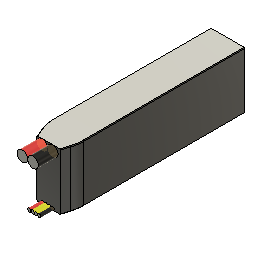
2024-11-05_development-hexapod-mounts (Autodesk Fusion 360 archive; units mm, degrees)
design "battery"
Autodesk Fusion 360 part; units mm, degrees
(part 1 of 2)
sketch "Sketch1" plane through (0, 0, 0) normal (0, 0, 1) x (1, 0, 0)
  line L0 (0, 0) -> (26, 0)
  line L1 (26, 0) -> (26, 137)
  line L2 (26, 137) -> (0, 137)
  line L3 (0, 137) -> (0, 0)
  dimension "d1" = 26
  dimension "d2" = 137
  constraint horizontal L0
  constraint vertical L1
  constraint horizontal L2
  constraint vertical L3
  constraint coincident L0.start L3.end
  measures "d1" distance of L0.start L0.end
  measures "d2" distance of L0.start L2.end
extrude "Extrude1" add sketch "Sketch1" along normal blind 43 makes body 1
sketch "Sketch2" plane through (0, 0, 0) normal (0, -1, 0) x (1, 0, 0)
  line L0 (0, 0) -> (26, 0)
  line L1 (26, 0) -> (26, 43)
  line L2 (26, 43) -> (0, 43)
  line L3 (0, 43) -> (0, 0)
  line L4 (21, 35) -> (5, 35) construction
  line L5 (5, 35) -> (5, 51) construction
  line L6 (5, 51) -> (21, 51) construction
  line L7 (21, 51) -> (21, 35) construction
  line L8 (21, 35) -> (5, 51) construction
  line L9 (5, 35) -> (21, 51) construction
  line L10 (13, 43) -> (5, 35) construction
  line L11 (13, 43) -> (21, 35) construction
  circle A0 centre (9, 39) radius 4
  circle A1 centre (17, 39) radius 4
  point P0 (13, 43)
  dimension "d5" = 16
  dimension "d6" = 16
  constraint horizontal L4
  constraint perpendicular L4 L5
  constraint parallel L4 L6
  constraint parallel L5 L7
  constraint coincident L8 P0
  constraint coincident L9 P0
  constraint midpoint L2 P0
  constraint coincident P0 L10.start
  constraint midpoint L10 A0.centre
  constraint tangent L2 A0
  constraint midpoint L11 A1.centre
  constraint tangent L2 A1
  measures "d5" distance of L5.end L6.end
  measures "d6" distance of L4.end L5.end
extrude "Extrude2" add sketch "Sketch2" along normal blind 15 separate body contours A0 | A1 makes body 2
sketch "Sketch3" plane through (0, 0, 0) normal (0, -1, 0) x (1, 0, 0)
  line L0 (0, 0) -> (26, 0)
  line L1 (26, 0) -> (26, 43)
  line L2 (26, 43) -> (0, 43)
  line L3 (0, 43) -> (0, 0)
  line L4 (18, 2.5) -> (8, 2.5) construction
  line L5 (8, 2.5) -> (8, -2.5) construction
  line L6 (8, -2.5) -> (18, -2.5) construction
  line L7 (18, -2.5) -> (18, 2.5) construction
  line L8 (18, 2.5) -> (8, -2.5) construction
  line L9 (8, 2.5) -> (18, -2.5) construction
  line L10 (8, 2.5) -> (8, 0)
  line L11 (8, 1.25) -> (9.25, 1.25) construction
  circle A0 centre (9.25, 1.25) radius 1.25
  circle A1 centre (11.75, 1.25) radius 1.25
  circle A2 centre (14.25, 1.25) radius 1.25
  circle A3 centre (16.75, 1.25) radius 1.25
  point P0 (13, 0)
  dimension "d9" = 10
  dimension "d10" = 5
  dimension "d11" = 1.25
  constraint horizontal L4
  constraint perpendicular L4 L5
  constraint parallel L4 L6
  constraint parallel L5 L7
  constraint coincident L8 P0
  constraint coincident L9 P0
  constraint midpoint L0 P0
  constraint midpoint L5 L10.end
  constraint midpoint L10 L11.start
  constraint perpendicular L5 L11
  constraint coincident L11.end A0.centre
  constraint tangent L4 A0
  measures "d9" distance of L5.end L6.end
  measures "d10" distance of L4.end L5.end
  measures "d11" distance of L11.start L11.end
extrude "Extrude3" add sketch "Sketch3" along normal blind 10 separate body contours A0 | A1 | A2 | A3 makes body 3
chamfer "Chamfer1" distance 3 distance2 10 1 edges at (26, 0, 21.5) measured on face at (8.6667, 0, 14.3333) on bodies 1
chamfer "Chamfer2" distance 12 distance2 5 1 edges at (0, 0, 21.5) measured on face at (0, 91.3333, 14.3333) on bodies 1
fillet "Fillet1" radius 30 2 edges at (0, 12, 21.5) (26, 10, 21.5) on bodies 1
chamfer "Chamfer3" distance 0.5 distance2 0.5 12 edges at (25.682, 10.0467, 0) (26, 75.7015, 0) (23.8674, 2.8913, 0) (0, 77.5, 0) (0.5826, 12.1165, 0) (3.6538, 3.2308, 0) (0.5826, 12.1165, 43) (0, 77.5, 43) (3.6538, 3.2308, 43) (26, 75.7015, 43) (23.8674, 2.8913, 43) (25.682, 10.0467, 43) 1 faces at (17.3333, 137, 14.3333) measured on face at (25.9843, 13.4317, 14.3333) measured on face at (26, 55.2687, 14.3333) measured on face at (23.5783, 1.9275, 14.3333) measured on face at (0, 97.3333, 14.3333) measured on face at (1.8284, 7.687, 28.6667) measured on face at (3.2051, 4.3077, 28.6667) measured on face at (1.8284, 7.687, 28.6667) measured on face at (17.3333, 56.4677, 43) measured on face at (3.2051, 4.3077, 28.6667) measured on face at (17.3333, 56.4677, 43) measured on face at (23.5783, 1.9275, 14.3333) measured on face at (25.9843, 13.4317, 14.3333) on bodies 1

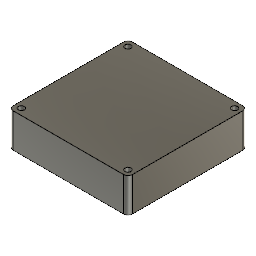
design "noctua_fan_80mm"
Autodesk Fusion 360 part; units mm, degrees
box "BoxPrimitive1" add length 80 width 80 height 23 placed x (0, -1, 0) y (1, 0, 0) z (0, 0, 1) at (0, 0, 0)
fillet "Fillet1" radius 3 4 edges at (0, -80, 11.5) (80, -80, 11.5) (80, 0, 11.5) (0, 0, 11.5)
sketch "Sketch2" plane through (0, 0, 23) normal (0, 0, 1) x (-1, 0, 0)
  arc A0 (-3, 0) -> (0, 3) centre (-3, 3) ccw
  line L0 (0, 3) -> (0, 77)
  arc A1 (0, 77) -> (-3, 80) centre (-3, 77) ccw
  line L1 (-3, 80) -> (-77, 80)
  arc A2 (-77, 80) -> (-80, 77) centre (-77, 77) ccw
  line L2 (-80, 77) -> (-80, 3)
  arc A3 (-80, 3) -> (-77, 0) centre (-77, 3) ccw
  line L3 (-77, 0) -> (-3, 0)
  circle A4 centre (-75.75, 75.75) radius 2
  circle A5 centre (-75.75, 4.25) radius 2
  circle A6 centre (-4.25, 75.75) radius 2
  circle A7 centre (-4.25, 4.25) radius 2
  dimension "d8" = 4
  dimension "d9" = 4
  dimension "d10" = 4
  dimension "d11" = 4
  dimension "d12" = 4.25
  dimension "d13" = 4.25
  dimension "d14" = 4.25
  dimension "d15" = 4.25
  dimension "d16" = 4.25
  dimension "d17" = 4.25
  dimension "d18" = 4.25
  dimension "d19" = 4.25
  measures "d8" diameter of A4
  measures "d9" diameter of A5
  measures "d10" diameter of A6
  measures "d11" diameter of A7
  measures "d12" distance of L1 A4.centre
  measures "d13" distance of L2 A4.centre
  measures "d14" distance of L3 A5.centre
  measures "d15" distance of L2 A5.centre
  measures "d16" distance of L3 A7.centre
  measures "d17" distance of L0 A7.centre
  measures "d18" distance of L1 A6.centre
  measures "d19" distance of L0 A6.centre
extrude "Extrude1" cut sketch "Sketch2" against normal blind 35 contours A4 | A5 | A6 | A7

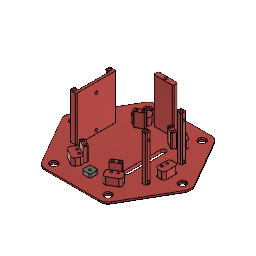
design "base"
Autodesk Fusion 360 part; units mm, degrees
sketch "Sketch1" plane through (0, 0, 0) normal (0, 0, 1) x (1, 0, 0)
  line L0 (130, 0) -> (65, 112.5833)
  line L1 (65, 112.5833) -> (-65, 112.5833)
  line L2 (-65, 112.5833) -> (-130, 0)
  line L3 (-130, 0) -> (-65, -112.5833)
  line L4 (-65, -112.5833) -> (65, -112.5833)
  line L5 (65, -112.5833) -> (130, 0)
  dimension "d1" = 130
  measures "d1" distance of L0.start origin
extrude "Extrude1" add sketch "Sketch1" along normal blind 6.5 makes body 1
fillet "Fillet1" radius 18 6 edges at (-130, 0, 3.25) (-65, -112.5833, 3.25) (65, -112.5833, 3.25) (130, 0, 3.25) (65, 112.5833, 3.25) (-65, 112.5833, 3.25) on bodies 1
chamfer "Chamfer2" distance 3.25 angle 45 12 edges at (0, -112.5833, 0) (63.6077, -110.1718, 0) (97.5, -56.2917, 0) (127.2154, 0, 0) (97.5, 56.2917, 0) (63.6077, 110.1718, 0) (0, 112.5833, 0) (-63.6077, 110.1718, 0) (-97.5, 56.2917, 0) (-127.2154, 0, 0) (-97.5, -56.2917, 0) (-63.6077, -110.1718, 0) on bodies 1
sketch "Sketch2" plane through (0, 0, 6.5) normal (0, 0, 1) x (-1, 0, 0)
  arc A0 (54.6077, -112.5833) -> (70.1962, -103.5833) centre (54.6077, -94.5833) ccw
  line L0 (70.1962, -103.5833) -> (124.8038, -9)
  arc A1 (124.8038, -9) -> (124.8038, 9) centre (109.2154, 0) ccw
  line L1 (124.8038, 9) -> (70.1962, 103.5833)
  line L2 (54.6077, 112.5833) -> (-54.6077, 112.5833)
  line L3 (-70.1962, 103.5833) -> (-124.8038, 9)
  arc A2 (-124.8038, 9) -> (-124.8038, -9) centre (-109.2154, 0) ccw
  line L4 (-124.8038, -9) -> (-70.1962, -103.5833)
  arc A3 (-70.1962, -103.5833) -> (-54.6077, -112.5833) centre (-54.6077, -94.5833) ccw
  line L5 (-54.6077, -112.5833) -> (54.6077, -112.5833)
  circle A4 centre (109.2154, 0) radius 7
  circle A5 centre (109.2154, 0) radius 6
  circle A6 centre (73.4654, -5) radius 2.25
  arc A7 (73.7154, 14.55) -> (68.7154, 9.55) centre (73.7154, 9.55) ccw
  line L6 (68.7154, 9.55) -> (68.7154, -9.55)
  circle A8 centre (73.4654, 5) radius 2.25
  line L7 (86.7154, 9.55) -> (86.7154, -9.55)
  line L8 (68.7154, 0) -> (86.7154, 0) construction
  arc A9 (68.7154, -9.55) -> (73.7154, -14.55) centre (73.7154, -9.55) ccw
  arc A10 (73.7154, 14.55) -> (68.7154, 9.55) centre (73.7154, 9.55) ccw
  line L9 (81.7154, 14.55) -> (73.7154, 14.55)
  line L10 (68.7154, 30.5204) -> (68.7154, -30.5204)
  line L11 (73.7154, -14.55) -> (81.7154, -14.55)
  line L12 (73.4654, 5) -> (68.7154, 5) construction
  line L13 (73.4654, -5) -> (68.7154, -5) construction
  line L14 (127.2154, 0) -> (-127.2154, 0) construction
  line L15 (0, -112.5833) -> (0, 112.5833) construction
  arc A11 (-124.8038, 9) -> (-124.8038, -9) centre (-109.2154, 0) ccw
  arc A12 (-70.1962, -103.5833) -> (-54.6077, -112.5833) centre (-54.6077, -94.5833) ccw
  arc A13 (54.6077, -112.5833) -> (70.1962, -103.5833) centre (54.6077, -94.5833) ccw
  arc A14 (81.7154, -14.55) -> (86.7154, -9.55) centre (81.7154, -9.55) ccw
  arc A15 (86.7154, 9.55) -> (81.7154, 14.55) centre (81.7154, 9.55) ccw
  circle A16 centre (32.4026, 66.1229) radius 2.25
  line L16 (26.0872, 64.2843) -> (42.6282, 54.7343)
  line L17 (34.3577, 59.5093) -> (43.3577, 75.0977) construction
  arc A17 (70.1962, 103.5833) -> (54.6077, 112.5833) centre (54.6077, 94.5833) ccw
  arc A18 (42.6282, 54.7343) -> (49.4584, 56.5644) centre (45.1282, 59.0644) ccw
  line L18 (41.0628, 61.1229) -> (38.6878, 57.0093) construction
  arc A19 (24.257, 71.1144) -> (26.0872, 64.2843) centre (28.5872, 68.6144) ccw
  line L19 (28.257, 78.0426) -> (24.257, 71.1144)
  circle A20 centre (41.0628, 61.1229) radius 2.25
  arc A21 (53.4584, 63.4926) -> (51.6282, 70.3227) centre (49.1282, 65.9926) ccw
  circle A22 centre (54.6077, 94.5833) radius 6
  circle A23 centre (54.6077, 94.5833) radius 7
  line L20 (32.4026, 66.1229) -> (30.0276, 62.0093) construction
  arc A24 (24.257, 71.1144) -> (26.0872, 64.2843) centre (28.5872, 68.6144) ccw
  line L21 (26.0872, 64.2843) -> (42.6282, 54.7343)
  line L22 (49.4584, 56.5644) -> (53.4584, 63.4926)
  line L23 (35.0872, 79.8727) -> (51.6282, 70.3227)
  arc A25 (35.0872, 79.8727) -> (28.257, 78.0426) centre (32.5872, 75.5426) ccw
  circle A26 centre (-41.0628, 61.1229) radius 2.25
  line L24 (-42.6282, 54.7343) -> (-26.0872, 64.2843)
  line L25 (-34.3577, 59.5093) -> (-43.3577, 75.0977) construction
  arc A27 (-54.6077, 112.5833) -> (-70.1962, 103.5833) centre (-54.6077, 94.5833) ccw
  arc A28 (-26.0872, 64.2843) -> (-24.257, 71.1144) centre (-28.5872, 68.6144) ccw
  line L26 (-32.4026, 66.1229) -> (-30.0276, 62.0093) construction
  arc A29 (-49.4584, 56.5644) -> (-42.6282, 54.7343) centre (-45.1282, 59.0644) ccw
  line L27 (-53.4584, 63.4926) -> (-49.4584, 56.5644)
  circle A30 centre (-32.4026, 66.1229) radius 2.25
  arc A31 (-28.257, 78.0426) -> (-35.0872, 79.8727) centre (-32.5872, 75.5426) ccw
  circle A32 centre (-54.6077, 94.5833) radius 6
  circle A33 centre (-54.6077, 94.5833) radius 7
  line L28 (-41.0628, 61.1229) -> (-38.6878, 57.0093) construction
  arc A34 (-49.4584, 56.5644) -> (-42.6282, 54.7343) centre (-45.1282, 59.0644) ccw
  line L29 (-42.6282, 54.7343) -> (-26.0872, 64.2843)
  line L30 (-24.257, 71.1144) -> (-28.257, 78.0426)
  line L31 (-51.6282, 70.3227) -> (-35.0872, 79.8727)
  arc A35 (-51.6282, 70.3227) -> (-53.4584, 63.4926) centre (-49.1282, 65.9926) ccw
  circle A36 centre (-73.4654, -5) radius 2.25
  line L32 (-68.7154, -9.55) -> (-68.7154, 9.55)
  line L33 (-68.7154, 0) -> (-86.7154, 0) construction
  arc A37 (-124.8038, 9) -> (-124.8038, -9) centre (-109.2154, 0) ccw
  arc A38 (-68.7154, 9.55) -> (-73.7154, 14.55) centre (-73.7154, 9.55) ccw
  line L34 (-73.4654, 5) -> (-68.7154, 5) construction
  arc A39 (-73.7154, -14.55) -> (-68.7154, -9.55) centre (-73.7154, -9.55) ccw
  line L35 (-81.7154, -14.55) -> (-73.7154, -14.55)
  circle A40 centre (-73.4654, 5) radius 2.25
  arc A41 (-81.7154, 14.55) -> (-86.7154, 9.55) centre (-81.7154, 9.55) ccw
  circle A42 centre (-109.2154, 0) radius 6
  circle A43 centre (-109.2154, 0) radius 7
  line L36 (-73.4654, -5) -> (-68.7154, -5) construction
  arc A44 (-73.7154, -14.55) -> (-68.7154, -9.55) centre (-73.7154, -9.55) ccw
  line L37 (-68.7154, -9.55) -> (-68.7154, 9.55)
  line L38 (-73.7154, 14.55) -> (-81.7154, 14.55)
  line L39 (-86.7154, -9.55) -> (-86.7154, 9.55)
  arc A45 (-86.7154, -9.55) -> (-81.7154, -14.55) centre (-81.7154, -9.55) ccw
  circle A46 centre (-32.4026, -66.1229) radius 2.25
  line L40 (-26.0872, -64.2843) -> (-42.6282, -54.7343)
  line L41 (-34.3577, -59.5093) -> (-43.3577, -75.0977) construction
  arc A47 (-70.1962, -103.5833) -> (-54.6077, -112.5833) centre (-54.6077, -94.5833) ccw
  arc A48 (-42.6282, -54.7343) -> (-49.4584, -56.5644) centre (-45.1282, -59.0644) ccw
  line L42 (-41.0628, -61.1229) -> (-38.6878, -57.0093) construction
  arc A49 (-24.257, -71.1144) -> (-26.0872, -64.2843) centre (-28.5872, -68.6144) ccw
  line L43 (-28.257, -78.0426) -> (-24.257, -71.1144)
  circle A50 centre (-41.0628, -61.1229) radius 2.25
  arc A51 (-53.4584, -63.4926) -> (-51.6282, -70.3227) centre (-49.1282, -65.9926) ccw
  circle A52 centre (-54.6077, -94.5833) radius 6
  circle A53 centre (-54.6077, -94.5833) radius 7
  line L44 (-32.4026, -66.1229) -> (-30.0276, -62.0093) construction
  arc A54 (-24.257, -71.1144) -> (-26.0872, -64.2843) centre (-28.5872, -68.6144) ccw
  line L45 (-26.0872, -64.2843) -> (-42.6282, -54.7343)
  line L46 (-49.4584, -56.5644) -> (-53.4584, -63.4926)
  line L47 (-35.0872, -79.8727) -> (-51.6282, -70.3227)
  arc A55 (-35.0872, -79.8727) -> (-28.257, -78.0426) centre (-32.5872, -75.5426) ccw
  circle A56 centre (41.0628, -61.1229) radius 2.25
  line L48 (42.6282, -54.7343) -> (26.0872, -64.2843)
  line L49 (34.3577, -59.5093) -> (43.3577, -75.0977) construction
  arc A57 (54.6077, -112.5833) -> (70.1962, -103.5833) centre (54.6077, -94.5833) ccw
  arc A58 (26.0872, -64.2843) -> (24.257, -71.1144) centre (28.5872, -68.6144) ccw
  line L50 (32.4026, -66.1229) -> (30.0276, -62.0093) construction
  arc A59 (49.4584, -56.5644) -> (42.6282, -54.7343) centre (45.1282, -59.0644) ccw
  line L51 (53.4584, -63.4926) -> (49.4584, -56.5644)
  circle A60 centre (32.4026, -66.1229) radius 2.25
  arc A61 (28.257, -78.0426) -> (35.0872, -79.8727) centre (32.5872, -75.5426) ccw
  circle A62 centre (54.6077, -94.5833) radius 6
  circle A63 centre (54.6077, -94.5833) radius 7
  line L52 (41.0628, -61.1229) -> (38.6878, -57.0093) construction
  arc A64 (49.4584, -56.5644) -> (42.6282, -54.7343) centre (45.1282, -59.0644) ccw
  line L53 (42.6282, -54.7343) -> (26.0872, -64.2843)
  line L54 (24.257, -71.1144) -> (28.257, -78.0426)
  line L55 (51.6282, -70.3227) -> (35.0872, -79.8727)
  arc A65 (51.6282, -70.3227) -> (53.4584, -63.4926) centre (49.1282, -65.9926) ccw
  circle A66 centre (73.4654, -5) radius 2.85
  circle A67 centre (73.4654, 5) radius 2.85
  circle A68 centre (41.0628, 61.1229) radius 2.85
  circle A69 centre (32.4026, 66.1229) radius 2.85
  circle A70 centre (-32.4026, 66.1229) radius 2.85
  circle A71 centre (-41.0628, 61.1229) radius 2.85
  circle A72 centre (-73.4654, 5) radius 2.85
  circle A73 centre (-73.4654, -5) radius 2.85
  circle A74 centre (-41.0628, -61.1229) radius 2.85
  circle A75 centre (-32.4026, -66.1229) radius 2.85
  circle A76 centre (32.4026, -66.1229) radius 2.85
  circle A77 centre (41.0628, -61.1229) radius 2.85
  line L56 (-75, -30.5) -> (-69, -30.5)
  line L57 (-67, -32.5) -> (-67, -38.5)
  line L58 (-69, -40.5) -> (-75, -40.5)
  line L59 (-77, -38.5) -> (-77, -32.5)
  line L60 (-77, -30.5) -> (-67, -40.5) construction
  line L61 (-67, -30.5) -> (-77, -40.5) construction
  line L62 (-75, 40.5) -> (-69, 40.5)
  line L63 (-67, 38.5) -> (-67, 32.5)
  line L64 (-69, 30.5) -> (-75, 30.5)
  line L65 (-77, 32.5) -> (-77, 38.5)
  line L66 (-77, 40.5) -> (-67, 30.5) construction
  line L67 (-67, 40.5) -> (-77, 30.5) construction
  line L68 (-72, -35.5) -> (-72, 13.37) construction
  line L69 (-72, 35.5) -> (-72, 30.8281) construction
  circle A78 centre (-72, 35.5) radius 2.85
  circle A79 centre (-72, -35.5) radius 2.85
  arc A80 (-67, -32.5) -> (-69, -30.5) centre (-69, -32.5) ccw
  arc A81 (-69, -40.5) -> (-67, -38.5) centre (-69, -38.5) ccw
  arc A82 (-75, -30.5) -> (-77, -32.5) centre (-75, -32.5) ccw
  arc A83 (-77, -38.5) -> (-75, -40.5) centre (-75, -38.5) ccw
  arc A84 (-69, 30.5) -> (-67, 32.5) centre (-69, 32.5) ccw
  arc A85 (-67, 38.5) -> (-69, 40.5) centre (-69, 38.5) ccw
  arc A86 (-75, 40.5) -> (-77, 38.5) centre (-75, 38.5) ccw
  arc A87 (-77, 32.5) -> (-75, 30.5) centre (-75, 32.5) ccw
  arc A88 (68.7154, -30.5204) -> (67, -32.5) centre (69, -32.5) ccw
  line L70 (77, -30.5) -> (67, -40.5) construction
  arc A89 (75, -40.5) -> (77, -38.5) centre (75, -38.5) ccw
  line L71 (69, -40.5) -> (75, -40.5)
  arc A90 (77, -32.5) -> (75, -30.5) centre (75, -32.5) ccw
  line L72 (77, -38.5) -> (77, -32.5)
  line L73 (67, -30.5) -> (77, -40.5) construction
  line L74 (67, -32.5) -> (67, -38.5)
  circle A91 centre (72, -35.5) radius 2.85
  line L75 (75, -30.5) -> (68.7154, -30.5)
  arc A92 (67, -38.5) -> (69, -40.5) centre (69, -38.5) ccw
  line L76 (68.7154, 30.5) -> (75, 30.5)
  arc A93 (77, 38.5) -> (75, 40.5) centre (75, 38.5) ccw
  line L77 (77, 32.5) -> (77, 38.5)
  line L78 (67, 38.5) -> (67, 32.5)
  line L79 (75, 40.5) -> (65.7154, 40.5)
  line L80 (77, 40.5) -> (67, 30.5) construction
  arc A94 (75, 30.5) -> (77, 32.5) centre (75, 32.5) ccw
  arc A95 (69, 40.5) -> (67, 38.5) centre (69, 38.5) ccw
  circle A96 centre (72, 35.5) radius 2.85
  arc A97 (67, 32.5) -> (68.7154, 30.5204) centre (69, 32.5) ccw
  line L81 (67, 40.5) -> (77, 30.5) construction
  line L82 (-29, 37.5) -> (-29, -37.5)
  line L83 (-39, -37.5) -> (-39, 37.5)
  line L84 (-39, 40.2042) -> (-29, -40) construction
  line L85 (-29, 40) -> (-39, -40.2042) construction
  line L86 (68.7154, 0) -> (68.7154, 5) construction
  line L87 (68.7154, 5) -> (65.7154, 5)
  line L88 (63.7154, 3) -> (63.7154, -3)
  line L89 (65.7154, -5) -> (68.7154, -5)
  line L90 (68.7154, -5) -> (68.7154, 5)
  line L91 (63.7154, -5) -> (68.7154, 5) construction
  line L92 (68.7154, -5) -> (63.7154, 5) construction
  arc A98 (63.7154, -3) -> (65.7154, -5) centre (65.7154, -3) ccw
  arc A99 (65.7154, 5) -> (63.7154, 3) centre (65.7154, 3) ccw
  line L93 (42.6282, -54.7343) -> (39.6282, -49.5381)
  line L94 (26.0872, -64.2843) -> (23.0872, -59.0881)
  line L95 (23.8192, -56.3561) -> (36.8962, -48.8061)
  circle A100 centre (36.6878, -53.5452) radius 2.35
  circle A101 centre (28.0276, -58.5452) radius 2.35
  line L96 (36.6878, -53.5452) -> (37.8628, -55.5803) construction
  line L97 (28.0276, -58.5452) -> (29.2026, -60.5803) construction
  arc A102 (39.6282, -49.5381) -> (36.8962, -48.8061) centre (37.8962, -50.5381) ccw
  arc A103 (23.8192, -56.3561) -> (23.0872, -59.0881) centre (24.8192, -58.0881) ccw
  line L98 (-42.6282, -54.7343) -> (-39.6282, -49.5381)
  line L99 (-42.6282, -54.7343) -> (-26.0872, -64.2843)
  arc A104 (-36.8962, -48.8061) -> (-39.6282, -49.5381) centre (-37.8962, -50.5381) ccw
  line L100 (-23.8192, -56.3561) -> (-36.8962, -48.8061)
  circle A105 centre (-36.6878, -53.5452) radius 2.35
  line L101 (-36.6878, -53.5452) -> (-37.8628, -55.5803) construction
  circle A106 centre (-28.0276, -58.5452) radius 2.35
  arc A107 (-23.0872, -59.0881) -> (-23.8192, -56.3561) centre (-24.8192, -58.0881) ccw
  line L102 (-26.0872, -64.2843) -> (-23.0872, -59.0881)
  line L103 (-28.0276, -58.5452) -> (-29.2026, -60.5803) construction
  line L104 (42.6282, 54.7343) -> (39.6282, 49.5381)
  line L105 (42.6282, 54.7343) -> (26.0872, 64.2843)
  arc A108 (36.8962, 48.8061) -> (39.6282, 49.5381) centre (37.8962, 50.5381) ccw
  line L106 (23.8192, 56.3561) -> (36.8962, 48.8061)
  circle A109 centre (36.6878, 53.5452) radius 2.35
  line L107 (36.6878, 53.5452) -> (37.8628, 55.5803) construction
  circle A110 centre (28.0276, 58.5452) radius 2.35
  line L108 (28.0276, 58.5452) -> (29.2026, 60.5803) construction
  arc A111 (23.0872, 59.0881) -> (23.8192, 56.3561) centre (24.8192, 58.0881) ccw
  line L109 (26.0872, 64.2843) -> (23.0872, 59.0881)
  line L110 (-26.0872, 64.2843) -> (-23.0872, 59.0881)
  arc A112 (-23.8192, 56.3561) -> (-23.0872, 59.0881) centre (-24.8192, 58.0881) ccw
  line L111 (-23.8192, 56.3561) -> (-36.8962, 48.8061)
  circle A113 centre (-28.0276, 58.5452) radius 2.35
  line L112 (-28.0276, 58.5452) -> (-29.2026, 60.5803) construction
  line L113 (-42.6282, 54.7343) -> (-26.0872, 64.2843)
  circle A114 centre (-36.6878, 53.5452) radius 2.35
  line L114 (-36.6878, 53.5452) -> (-37.8628, 55.5803) construction
  arc A115 (-39.6282, 49.5381) -> (-36.8962, 48.8061) centre (-37.8962, 50.5381) ccw
  line L115 (-42.6282, 54.7343) -> (-39.6282, 49.5381)
  arc A116 (-39, -37.5) -> (-29, -37.5) centre (-34, -37.5) ccw
  arc A117 (-29, 37.5) -> (-39, 37.5) centre (-34, 37.5) ccw
  line L116 (63.7154, 3) -> (63.7154, 38.5)
  line L117 (63.7154, -1.8213) -> (63.7154, -38.5)
  line L118 (69, -40.5) -> (65.7154, -40.5)
  arc A118 (65.7154, 40.5) -> (63.7154, 38.5) centre (65.7154, 38.5) ccw
  arc A119 (63.7154, -38.5) -> (65.7154, -40.5) centre (65.7154, -38.5) ccw
  line L119 (-6, 84.2496) -> (6.5, 84.2496)
  line L120 (8.5, 82.2496) -> (8.5, 69.7496)
  line L121 (6.5, 67.7496) -> (-6, 67.7496)
  line L122 (-8, 69.7496) -> (-8, 82.2496)
  line L123 (-8, 84.2496) -> (8.5, 67.7496) construction
  line L124 (8.5, 84.2496) -> (-8, 67.7496) construction
  arc A120 (6.5, 67.7496) -> (8.5, 69.7496) centre (6.5, 69.7496) ccw
  arc A121 (8.5, 82.2496) -> (6.5, 84.2496) centre (6.5, 82.2496) ccw
  arc A122 (-6, 84.2496) -> (-8, 82.2496) centre (-6, 82.2496) ccw
  arc A123 (-8, 69.7496) -> (-6, 67.7496) centre (-6, 69.7496) ccw
  circle A124 centre (0.25, 75.9996) radius 2.25
  circle A125 centre (0.25, 75.9996) radius 2.85
  circle A126 centre (0, -76) radius 2.85
  line L125 (-18, -71) -> (18, -71)
  line L126 (20, -73) -> (20, -79)
  line L127 (18, -81) -> (-18, -81)
  line L128 (-20, -79) -> (-20, -73)
  line L129 (-20, -71) -> (20, -81) construction
  line L130 (20, -71) -> (-20, -81) construction
  arc A127 (18, -81) -> (20, -79) centre (18, -79) ccw
  arc A128 (20, -73) -> (18, -71) centre (18, -73) ccw
  arc A129 (-18, -71) -> (-20, -73) centre (-18, -73) ccw
  arc A130 (-20, -79) -> (-18, -81) centre (-18, -79) ccw
  point P0 (63.6077, 110.1718)
  point P1 (-63.6077, 110.1718)
  point P2 (-127.2154, 0)
  point P3 (-63.6077, -110.1718)
  point P4 (63.6077, -110.1718)
  point P5 (-72, -35.5)
  point P6 (-72, 35.5)
  point P7 (72, -35.5)
  point P8 (72, -35.5)
  point P9 (72, 35.5)
  point P10 (72, 35.5)
  point P11 (-33.9873, 0)
  point P12 (38.6282, -47.8061)
  point P13 (22.0872, -57.3561)
  point P14 (0, 76)
  point P15 (0, 72)
  point P16 (0.25, 75.9996)
  point P17 (0, -76)
  dimension "d8" = 14
  dimension "d9" = 12
  dimension "d10" = 18
  dimension "d11" = 9.55
  dimension "d12" = 9.55
  dimension "d13" = 4.75
  dimension "d14" = 4.75
  dimension "d15" = 29.1
  dimension "d16" = 40.5
  dimension "d30" = 5
  dimension "d33" = 4.5
  dimension "d34" = 4.5
  dimension "d35" = 5.7
  dimension "d36" = 5.7
  dimension "d43" = 10
  dimension "d44" = 10
  dimension "d45" = 10
  dimension "d46" = 10
  dimension "d49" = 72
  dimension "d50" = 5.7
  dimension "d51" = 5.7
  dimension "d53" = 2
  dimension "d75" = 35.5
  dimension "d76" = 35.5
  dimension "d78" = 80
  dimension "d79" = 29
  dimension "d84" = 5
  dimension "d85" = 5
  dimension "d86" = 10
  dimension "d87" = 2
  dimension "d98" = 8
  dimension "d99" = 8
  dimension "d100" = 4.7
  dimension "d101" = 4.7
  dimension "d102" = 4
  dimension "d103" = 4
  dimension "d104" = 2
  dimension "d135" = 10
  dimension "d136" = 2
  dimension "d137" = 2
  dimension "d164" = 16.5
  dimension "d165" = 16.5
  dimension "d166" = 2
  dimension "d170" = 76
  dimension "d171" = 4.5
  dimension "d172" = 5.7
  dimension "d173" = 5.7
  dimension "d174" = 76
  dimension "d175" = 40
  dimension "d176" = 10
  dimension "d177" = 2
  constraint concentric A1 A4
  constraint concentric A4 A5
  constraint coincident A7.end L6.start
  constraint coincident L6.end A9.start
  constraint tangent A10 L10
  constraint perpendicular L8 L10
  constraint coincident A9.end L11.start
  constraint coincident A7.start A10.start
  constraint coincident L8.end L7
  constraint parallel L9 L11
  constraint parallel L6 L7
  constraint coincident A8.centre L12.start
  constraint coincident L10 L12.end
  constraint perpendicular L10 L12
  constraint coincident A6.centre L13.start
  constraint coincident L10 L13.end
  constraint perpendicular L10 L13
  constraint midpoint A1 L14.start
  constraint midpoint A2 P2
  constraint midpoint L5 L15.start
  constraint midpoint L2 L15.end
  constraint collinear L8 L14
  constraint tangent L11 A14
  constraint tangent L7 A14
  constraint tangent L7 A15
  constraint tangent L9 A15
  constraint equal A14 A15
  constraint concentric A6 A66
  constraint horizontal L56
  constraint perpendicular L56 L57
  constraint parallel L56 L58
  constraint parallel L57 L59
  constraint coincident L60 P5
  constraint coincident L61 P5
  constraint horizontal L62
  constraint perpendicular L62 L63
  constraint parallel L62 L64
  constraint parallel L63 L65
  constraint coincident L66 P6
  constraint coincident L67 P6
  constraint coincident P5 L68.start
  constraint perpendicular L56 L68
  constraint coincident P6 L69.start
  constraint perpendicular L64 L69
  constraint collinear L68 L69
  constraint coincident L61.start L57
  constraint coincident L61.start L56
  constraint tangent L57 A80
  constraint tangent L56 A80
  constraint coincident L60.end L58
  constraint coincident L60.end L57
  constraint tangent L58 A81
  constraint tangent L57 A81
  constraint equal A80 A81
  constraint coincident L60.start L59
  constraint coincident L60.start L56
  constraint tangent L59 A82
  constraint tangent L56 A82
  constraint equal A80 A82
  constraint coincident L61.end L58
  constraint coincident L61.end L59
  constraint tangent L58 A83
  constraint tangent L59 A83
  constraint equal A80 A83
  constraint coincident L66.end L64
  constraint coincident L66.end L63
  constraint tangent L64 A84
  constraint tangent L63 A84
  constraint equal A80 A84
  constraint coincident L67.start L63
  constraint coincident L67.start L62
  constraint tangent L63 A85
  constraint tangent L62 A85
  constraint equal A80 A85
  constraint coincident L66.start L65
  constraint coincident L66.start L62
  constraint tangent L65 A86
  constraint tangent L62 A86
  constraint equal A80 A86
  constraint coincident L67.end L65
  constraint coincident L67.end L64
  constraint tangent L65 A87
  constraint tangent L64 A87
  constraint equal A80 A87
  constraint symmetric L15 L60.start L70.start
  constraint symmetric L15 L61.start L73.start
  constraint symmetric L15 L60.end L70.end
  constraint symmetric L15 L61.end L73.end
  constraint symmetric L15 P5 P8
  constraint symmetric L15 L66.start L80.start
  constraint symmetric L15 P6 P10
  constraint symmetric L15 A78 A96
  constraint symmetric L15 A79 A91
  constraint symmetric L15 L57.start A88.end
  constraint symmetric L15 A80 A88
  constraint symmetric L15 L58.start L71.start
  constraint symmetric L15 L57.end L74.end
  constraint symmetric L15 A81 A92
  constraint symmetric L15 L59.end A90.start
  constraint symmetric L15 L56.start A90.end
  constraint symmetric L15 A82 A90
  constraint symmetric L15 L58.end A89.start
  constraint symmetric L15 L59.start A89.end
  constraint symmetric L15 A83 A89
  constraint symmetric L15 L63.end L78.end
  constraint symmetric L15 A84 A97
  constraint symmetric L15 L63.start L78.start
  constraint symmetric L15 L62.end A95.start
  constraint symmetric L15 A85 A95
  constraint symmetric L15 L65.end A93.start
  constraint symmetric L15 L62.start A93.end
  constraint symmetric L15 A86 A93
  constraint symmetric L15 L65.start L77.start
  constraint symmetric L15 L64.end L76.end
  constraint symmetric L15 A87 A94
  constraint parallel L82 L83
  constraint coincident L84 P11
  constraint coincident L85 P11
  constraint coincident L14 P11
  constraint coincident L84.end L82
  constraint coincident L85.end L83
  constraint coincident L85.start L82
  constraint coincident L84.start L83
  constraint perpendicular L8 L86
  constraint horizontal L87
  constraint vertical L88
  constraint horizontal L89
  constraint vertical L90
  constraint coincident L91.start L89
  constraint coincident L91.start L88
  constraint tangent L89 A98
  constraint tangent L88 A98
  constraint coincident L92.end L88
  constraint coincident L92.end L87
  constraint tangent L88 A99
  constraint tangent L87 A99
  constraint equal A98 A99
  constraint perpendicular L48 L93
  constraint perpendicular L48 L94
  constraint coincident A100.centre L96.start
  constraint coincident A100 L96.end
  constraint perpendicular L48 L96
  constraint coincident A101.centre L97.start
  constraint coincident A101 L97.end
  constraint perpendicular L48 L97
  constraint collinear L52 L96
  constraint collinear L50 L97
  constraint coincident P12 L93
  constraint coincident P12 L95
  constraint tangent L93 A102
  constraint tangent L95 A102
  constraint coincident P13 L95
  constraint coincident P13 L94
  constraint tangent L95 A103
  constraint tangent L94 A103
  constraint equal A102 A103
  constraint symmetric L15 L48.start L40.end
  constraint symmetric L15 L48.end L40.start
  constraint symmetric L15 A100 A105
  constraint symmetric L15 A101 A106
  constraint symmetric L15 A100.centre A105.centre
  constraint symmetric L15 L96.end L101.end
  constraint symmetric L15 A101.centre A106.centre
  constraint symmetric L15 L97.end L103.end
  constraint symmetric L15 L93.end L98.end
  constraint symmetric L15 L95.end A104.start
  constraint symmetric L15 A102 A104
  constraint symmetric L15 L95.start L100.start
  constraint symmetric L15 L94.end A107.start
  constraint symmetric L15 A103 A107
  constraint symmetric L14 L48.start L16.end
  constraint symmetric L14 L48.end L16.start
  constraint symmetric L14 A100 A109
  constraint symmetric L14 A101 A110
  constraint symmetric L14 A100.centre A109.centre
  constraint symmetric L14 L96.end L107.end
  constraint symmetric L14 A101.centre A110.centre
  constraint symmetric L14 L97.end L108.end
  constraint symmetric L14 L93.end L104.end
  constraint symmetric L14 L95.end A108.start
  constraint symmetric L14 A102 A108
  constraint symmetric L14 L95.start L106.start
  constraint symmetric L14 L94.end A111.start
  constraint symmetric L14 A103 A111
  constraint symmetric L14 L40.end L24.start
  constraint symmetric L14 L98.end A115.start
  constraint symmetric L14 L40.start L24.end
  constraint symmetric L14 A104.start L111.end
  constraint symmetric L14 A104 A115
  constraint symmetric L14 L100.start A112.start
  constraint symmetric L14 A105 A114
  constraint symmetric L14 A105.centre A114.centre
  constraint symmetric L14 L101.end L114.end
  constraint symmetric L14 A106 A113
  constraint symmetric L14 A107.start L110.end
  constraint symmetric L14 A107 A112
  constraint symmetric L14 A106.centre A113.centre
  constraint symmetric L14 L103.end L112.end
  constraint tangent L83 A116
  constraint tangent L83 A117
  constraint tangent A99 L116
  constraint coincident L88 L117.start
  constraint parallel L88 L117
  constraint tangent A92 L118
  constraint coincident A95.start L79
  constraint coincident L81.start L79
  constraint tangent L79 A118
  constraint tangent L116 A118
  constraint tangent L118 A119
  constraint tangent L117 A119
  constraint coincident L8.start L10
  constraint coincident A7.end L10
  constraint coincident L6.end L10
  constraint horizontal L119
  constraint perpendicular L119 L120
  constraint parallel L119 L121
  constraint parallel L120 L122
  constraint coincident L123 P16
  constraint coincident L124 P16
  constraint coincident L123.end L121
  constraint coincident L123.end L120
  constraint tangent L121 A120
  constraint tangent L120 A120
  constraint coincident L124.start L120
  constraint coincident L124.start L119
  constraint tangent L120 A121
  constraint tangent L119 A121
  constraint equal A120 A121
  constraint coincident L123.start L119
  constraint coincident L123.start L122
  constraint tangent L119 A122
  constraint tangent L122 A122
  constraint equal A120 A122
  constraint coincident L124.end L122
  constraint coincident L124.end L121
  constraint tangent L122 A123
  constraint tangent L121 A123
  constraint equal A120 A123
  constraint coincident P16 A124.centre
  constraint concentric A124 A125
  constraint coincident L15 P17
  constraint horizontal L125
  constraint perpendicular L125 L126
  constraint parallel L125 L127
  constraint parallel L126 L128
  constraint coincident L129 P17
  constraint coincident L130 P17
  constraint coincident P17 A126.centre
  constraint coincident L129.end L127
  constraint coincident L129.end L126
  constraint tangent L127 A127
  constraint tangent L126 A127
  constraint coincident L130.start L126
  constraint coincident L130.start L125
  constraint tangent L126 A128
  constraint tangent L125 A128
  constraint equal A127 A128
  constraint coincident L129.start L125
  constraint coincident L129.start L128
  constraint tangent L125 A129
  constraint tangent L128 A129
  constraint equal A127 A129
  constraint coincident L130.end L128
  constraint coincident L130.end L127
  constraint tangent L128 A130
  constraint tangent L127 A130
  constraint equal A127 A130
  measures "d8" diameter of A4
  measures "d9" diameter of A5
  measures "d10" distance of L8.end L8.start
  measures "d11" distance of A8.centre L9
  measures "d12" distance of A6.centre L11
  measures "d13" distance of A6.centre L10
  measures "d14" distance of A8.centre L10
  measures "d15" distance of L9 L11
  measures "d16" distance of A1.centre L10
  measures "d30" radius of A14
  measures "d33" diameter of A6
  measures "d34" diameter of A8
  measures "d35" diameter of A66
  measures "d36" diameter of A67
  measures "d43" distance of L60.end L61.end
  measures "d44" distance of L61.start L60.end
  measures "d45" distance of L66.end L67.end
  measures "d46" distance of L67.start L66.end
  measures "d49" distance of L15 P6
  measures "d50" diameter of A78
  measures "d51" diameter of A79
  measures "d53" radius of A80
  measures "d75" distance of L14 P5
  measures "d76" distance of L14 P6
  measures "d78" distance of L85.start L84.end
  measures "d79" distance of origin L82
  measures "d84" distance of L8.start L12.end
  measures "d85" distance of L12.end L92.end
  measures "d86" distance of L12.end L13.end
  measures "d87" radius of A98
  measures "d98" distance of L48.start P12
  measures "d99" distance of L48.end P13
  measures "d100" diameter of A100
  measures "d101" diameter of A101
  measures "d102" distance of L95 A100.centre
  measures "d103" distance of L95 A101.centre
  measures "d104" radius of A102
  measures "d135" distance of L82 L83
  measures "d136" radius of A118
  measures "d137" radius of A119
  measures "d164" distance of L123.end L124.end
  measures "d165" distance of L124.start L123.end
  measures "d166" radius of A120
  measures "d170" distance of origin P16
  measures "d171" diameter of A124
  measures "d172" diameter of A125
  measures "d173" diameter of A126
  measures "d174" distance of origin P17
  measures "d175" distance of L129.end L130.end
  measures "d176" distance of L130.start L129.end
  measures "d177" radius of A127
extrude "Extrude2" cut sketch "Sketch2" against normal blind 6.5 contours A5 | A22 | A32 | A42 | A52 | A62 bodies 1
extrude "Extrude3" cut sketch "Sketch2" along normal blind 4.25 from surface at -6.5 contours A4 | A23 | A33 | A43 | A53 | A63 bodies 1
fillet "Fillet5" radius 0.5 6 edges at (-102.6891, 2.5313, 4.25) (-53.5367, -87.6657, 4.25) (49.1524, -90.197, 4.25) (-49.1524, 90.197, 4.25) (53.5367, 87.6657, 4.25) (102.6891, -2.5313, 4.25) on bodies 1
chamfer "Chamfer1" distance 1.5 angle 45 6 edges at (-103.6214, -2.1697, 6.5) (-53.6897, 88.6539, 6.5) (-49.9317, -90.8236, 6.5) (53.6897, -88.6539, 6.5) (49.9317, 90.8236, 6.5) (103.6214, 2.1697, 6.5) on bodies 1
extrude "Extrude4" add sketch "Sketch2" along normal blind 14.5 contours A7 L6 L7 A9 A10 L9 L10 L11 A14 A15 L90 | L16 A18 A19 L19 A21 A24 L21 L22 L23 A25 L105 | L24 A28 A29 L27 A31 A34 L29 L30 L31 A35 L113 | L32 A38 A39 L35 A41 A44 L37 L38 L39 A45 | L40 A48 A49 L43 A51 A54 L45 L46 L47 A55 L99 | L48 A58 A59 L51 A61 A64 L53 L54 L55 A65 | A66 | A67 | A68 | A69 | A70 | A71 | A72 | A73 | A74 | A75 | A76 | A77 bodies 1
extrude "Extrude6" cut sketch "Sketch2" against normal blind 6.5 contours A6 | A8 | A16 | A20 | A26 | A30 | A36 | A40 | A46 | A50 | A56 | A60 | A66 | A67 | A68 | A69 | A70 | A71 | A72 | A73 | A74 | A75 | A76 | A77 bodies 1
extrude "Extrude7" add sketch "Sketch2" along normal blind 90 contours L6 L10 L78 L79 A95 A97 L87 A99 L116 A118 | L6 L10 L87 L88 L89 L90 A98 A99 L117 | L10 L76 A93 L77 L78 L79 A94 A95 A97 | L6 L10 A88 L74 A92 L89 A98 L117 L118 A119 | L10 A88 A89 L71 A90 L72 L74 L75 A92 | L56 L57 L58 L59 A80 A81 A82 A83 | L62 L63 L64 L65 A84 A85 A86 A87 | A78 | A79 | A91 | A96 | A126 | L125 L126 L127 L128 A127 A128 A129 A130 bodies 1
extrude "Extrude8" cut sketch "Sketch2" against normal blind 5 from surface at 90 contours A78 | A79 | A91 | A96 | A126 bodies 1
extrude "Extrude20" add sketch "Sketch2" along normal blind 7 separate body contours L119 L120 L121 L122 A120 A121 A122 A123 | A125 makes body 2
extrude "Extrude21" cut sketch "Sketch2" against normal blind 6.5 from surface at -1.5 contours A124 | A125 bodies 1
extrude "Extrude22" cut sketch "Sketch2" against normal blind 6.5 contours A124 bodies 1
sketch "Sketch4" plane through (77, 0, 0) normal (1, 0, 0) x (0, 1, 0)
  line L0 (32.5, 6.5) -> (38.5, 6.5)
  line L1 (38.5, 6.5) -> (38.5, 96.5)
  line L2 (38.5, 96.5) -> (32.5, 96.5)
  line L3 (32.5, 96.5) -> (32.5, 6.5)
  circle A0 centre (-35.5, 82.5) radius 2.75
  circle A1 centre (-35.5, 82.5) radius 1.75
  line L4 (-32.5, 6.5) -> (-38.5, 6.5) construction
  line L5 (38.5, 6.5) -> (32.5, 6.5) construction
  line L6 (-35.5, 6.5) -> (-35.5, 81) construction
  line L7 (-35.5, 82.5) -> (-35.5, 79.75) construction
  circle A2 centre (-35.5, 10.5) radius 2.75
  circle A3 centre (-35.5, 10.5) radius 1.75
  line L8 (0, 2.5) -> (0, 20) construction
  circle A4 centre (35.5, 10.5) radius 1.75
  circle A5 centre (35.5, 10.5) radius 2.75
  circle A6 centre (35.5, 82.5) radius 1.75
  line L9 (35.5, 6.5) -> (35.5, 81) construction
  line L10 (32.5, 6.5) -> (38.5, 6.5) construction
  line L11 (35.5, 82.5) -> (35.5, 79.75) construction
  circle A7 centre (35.5, 82.5) radius 2.75
  dimension "d59" = 5.5
  dimension "d60" = 3.5
  dimension "d62" = 76
  dimension "d63" = 5.5
  dimension "d64" = 4
  dimension "d65" = 3.5
  constraint concentric A0 A1
  constraint midpoint L4 L6.start
  constraint perpendicular L4 L6
  constraint coincident A0.centre A1.centre
  constraint coincident A0 L7.end
  constraint vertical L7
  constraint collinear L6 L7
  constraint coincident L6 A2.centre
  constraint concentric A2 A3
  constraint symmetric A0 L8 A7
  constraint symmetric A1 L8 A6
  constraint symmetric L4.start L8 L0.start
  constraint symmetric L4.end L8 L0.end
  constraint symmetric L6.start L8 L9.start
  constraint symmetric L6.end L8 L9.end
  constraint symmetric A0.centre L8 A6.centre
  constraint symmetric L7.end L8 L11.end
  constraint symmetric A2 L8 A5
  constraint symmetric A3 L8 A4
  measures "d59" diameter of A0
  measures "d60" diameter of A1
  measures "d62" distance of A0.centre L6.start
  measures "d63" diameter of A2
  measures "d64" distance of L4 A2.centre
  measures "d65" diameter of A3
extrude "Extrude9" cut sketch "Sketch4" against normal blind 5 contours A0 | A1 | A2 | A3 | A4 | A5 | A6 | A7 bodies 1
extrude "Extrude10" cut sketch "Sketch4" against normal up to surface (10 mm away) contours A1 | A3 | A4 | A6 bodies 1
extrude "Extrude11" cut sketch "Sketch2" against normal blind 6.5 contours L82 L83 A116 A117 bodies 1
sketch "Sketch5" plane through (-63.7154, 0, 0) normal (1, 0, 0) x (0, 1, 0)
  line L0 (-38.5, 6.5) -> (38.5, 6.5)
  line L1 (38.5, 92.5) -> (-38.5, 92.5)
  circle A0 centre (0, 77.5) radius 2.85
  circle A1 centre (0, 12.5) radius 2.85
  line L2 (0, 12.5) -> (0, 9.65) construction
  line L3 (0, 77.5) -> (0, 74.65) construction
  line L4 (38.5, 6.5) -> (-38.5, 6.5) construction
  line L5 (0, 6.5) -> (0, 92.5) construction
  line L6 (38.5, 6.5) -> (38.5, 92.5)
  line L7 (-38.5, 92.5) -> (-38.5, 6.5)
  line L8 (-38.5, 6.5) -> (38.5, 6.5)
  line L9 (38.5, 96.5) -> (-38.5, 96.5)
  line L10 (38.5, 6.5) -> (38.5, 96.5)
  line L11 (-38.5, 96.5) -> (-38.5, 6.5)
  dimension "d90" = 5.7
  dimension "d91" = 5.7
  dimension "d92" = 6
  dimension "d93" = 71
  constraint coincident A1.centre L2.start
  constraint coincident A1 L2.end
  constraint coincident A0.centre L3.start
  constraint coincident A0 L3.end
  constraint midpoint L0 L5.start
  constraint midpoint L1 L5.end
  constraint collinear L3 L5
  constraint collinear L2 L5
  measures "d90" diameter of A0
  measures "d91" diameter of A1
  measures "d92" distance of L0 A1.centre
  measures "d93" distance of A0.centre L4
extrude "Extrude13" cut sketch "Sketch5" against normal blind 15 contours A0 | A1 bodies 1
extrude "Extrude14" add sketch "Sketch2" along normal blind 28 contours L16 L21 L104 L105 A108 L106 A111 L109 | L24 L29 L110 A112 L111 L113 A115 L115 | L40 L45 L98 L99 A104 L100 A107 L102 | L48 L53 L93 L94 L95 A102 A103 | A100 | A101 | A105 | A106 | A109 | A110 | A113 | A114 bodies 1
extrude "Extrude15" cut sketch "Sketch2" against normal blind 5 from surface at 28 contours A100 | A101 | A105 | A106 | A109 | A110 | A113 | A114 bodies 1